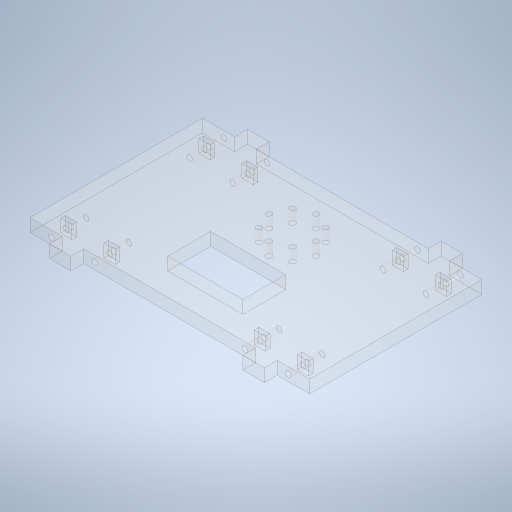
# Autodesk Inventor part: frame_waist_frames_linker1
Saved by Autodesk Inventor 2024 (Build 280153000, 153)
## iProperties
Created: 2024-09-07
Part Number: frame_waist_frames_linker1
Material: PMMA 플라스틱
Document SubType Name: Modeling
Designer: jmha0
Density: 1.188 g/cm^3
Appearance: 폴리카보네이트 - 선명
Author: jmha0
Autodesk Inventor part; units mm, degrees
ref_plane "YZ Plane" through (0, 0, 0) normal (1, 0, 0) x (0, 1, 0)
ref_plane "XZ Plane" through (0, 0, 0) normal (0, 1, 0) x (-1, 0, 0)
ref_plane "XY Plane" through (0, 0, 0) normal (0, 0, 1) x (1, 0, 0)
sketch "스케치1" plane through (0, 0, 0) normal (0, 1, 0) x (-1, 0, 0)
  circle A0 centre (21.5232, -91.3038) radius 1.65
  circle A1 centre (37.0796, -75.7475) radius 1.65
  circle A2 centre (29.3014, -72.5257) radius 1.65
  circle A3 centre (29.3014, -94.5257) radius 1.65
  circle A4 centre (18.3014, -83.5257) radius 1.65
  circle A5 centre (40.3014, -83.5257) radius 1.65
  circle A6 centre (21.5232, -75.7475) radius 1.65
  circle A7 centre (37.0796, -91.3038) radius 1.65
  line L0 (-35.8986, -112.7138) -> (94.5014, -112.7138)
  line L1 (94.5014, -112.7138) -> (94.5014, -20.3138)
  line L2 (94.5014, -20.3138) -> (-35.8986, -20.3138)
  line L3 (-35.8986, -20.3138) -> (-35.8986, -112.7138)
  circle A8 centre (-5.7486, -109.7138) radius 1.45
  circle A9 centre (-25.8486, -109.7138) radius 1.45
  circle A10 centre (-25.8486, -23.3138) radius 1.45
  circle A11 centre (-5.7486, -23.3138) radius 1.45
  circle A12 centre (64.3514, -23.3138) radius 1.45
  circle A13 centre (84.4514, -23.3138) radius 1.45
  circle A14 centre (84.4514, -109.7138) radius 1.45
  circle A15 centre (64.3514, -109.7138) radius 1.45
  line L4 (94.5014, -20.3138) -> (-35.8986, -20.3138)
  line L5 (-35.8986, -20.3138) -> (-35.8986, -26.3138)
  line L6 (-35.8986, -26.3138) -> (94.5014, -26.3138)
  line L7 (94.5014, -26.3138) -> (94.5014, -20.3138)
  line L8 (94.5014, -112.7138) -> (-35.8986, -112.7138)
  line L9 (-35.8986, -112.7138) -> (-35.8986, -106.7138)
  line L10 (-35.8986, -106.7138) -> (94.5014, -106.7138)
  line L11 (94.5014, -106.7138) -> (94.5014, -112.7138)
  circle A16 centre (29.3014, -94.5257) radius 1.35
  circle A17 centre (21.5232, -91.3038) radius 1.35
  circle A18 centre (18.3014, -83.5257) radius 1.35
  circle A19 centre (21.5232, -75.7475) radius 1.35
  circle A20 centre (29.3014, -72.5257) radius 1.35
  circle A21 centre (37.0796, -75.7475) radius 1.35
  circle A22 centre (40.3014, -83.5257) radius 1.35
  circle A23 centre (37.0796, -91.3038) radius 1.35
  point P0 (0, 0)
  point P1 (81.123, -83.5257)
  dimension "d0" = 6
  dimension "d1" = 6
  dimension "d16" = 2.7
  dimension "d17" = 2.7
  dimension "d18" = 2.7
  dimension "d19" = 2.7
  dimension "d20" = 2.7
  dimension "d21" = 2.7
  dimension "d22" = 2.7
  dimension "d23" = 2.7
  constraints: 24 centre point, 24 end point, 8 coincident, 4 parallel, 2 horizontal, 2 perpendicular, 2 point on line
  measures "d0" distance of L5.end L4.end
  measures "d1" distance of L8.end L9.end
  measures "d16" diameter of A16
  measures "d17" diameter of A17
  measures "d18" diameter of A18
  measures "d19" diameter of A19
  measures "d20" diameter of A20
  measures "d21" diameter of A21
  measures "d22" diameter of A22
  measures "d23" diameter of A23
extrude "돌출1" add sketch "스케치1" along normal blind 6 contours A0 | A1 | A2 | A3 | A4 | A5 | A6 | A7 | L3 L6 L1 L10
sketch "스케치2" plane through (-94.5014, 0, -26.3138) normal (0, 0, 1) x (1, 0, 0)
  line L0 (0, 0) -> (130.4, 0) projected
  line L1 (130.4, 0) -> (130.4, 6) projected
  line L2 (0, 6) -> (130.4, 6) projected
  line L3 (0, 0) -> (0, 6) projected
  line L4 (0, 6) -> (10.05, 6)
  line L5 (10.05, 6) -> (30.15, 6)
  line L6 (130.4, 6) -> (120.35, 6)
  line L7 (130.4, 6) -> (0, 6) projected
  line L8 (120.35, 6) -> (100.25, 6)
  circle A0 centre (10.05, 3) radius 1.35
  circle A1 centre (30.15, 3) radius 1.35
  circle A2 centre (100.25, 3) radius 1.35
  circle A3 centre (120.35, 3) radius 1.35
  point P0 (94.5014, 0)
  dimension "d4" = 10.05
  dimension "d5" = 20.1
  dimension "d6" = 10.05
  dimension "d7" = 20.1
  dimension "d8" = 2.7
  dimension "d9" = 2.7
  dimension "d10" = 2.7
  dimension "d11" = 2.7
  constraints: 8 end point, 4 centre point, 4 point on line
  measures "d4" distance of L2.start L4.end
  measures "d5" distance of L4.end L5.end
  measures "d6" distance of L1.end L6.end
  measures "d7" distance of L6.end L8.end
  measures "d8" diameter of A0
  measures "d9" diameter of A1
  measures "d10" diameter of A2
  measures "d11" diameter of A3
extrude "돌출2" cut sketch "스케치2" against normal blind 16 contours A0 | A1 | A2 | A3
sketch "스케치3" plane through (35.8986, 0, -106.7138) normal (0, 0, -1) x (-1, 0, 0)
  circle A0 centre (30.15, 3) radius 1.35 projected
  circle A1 centre (100.25, 3) radius 1.35 projected
  point P0 (35.8986, 0)
extrude "돌출3" cut sketch "스케치3" against normal blind 16
sketch "스케치4" plane through (35.8986, 0, -106.7138) normal (0, 0, -1) x (-1, 0, 0)
  circle A0 centre (10.05, 3) radius 1.35 projected
  circle A1 centre (120.35, 3) radius 1.35 projected
  point P0 (35.8986, 0)
extrude "돌출4" cut sketch "스케치4" against normal blind 16
sketch "스케치5" plane through (0, 6, 0) normal (0, 1, 0) x (1, 0, 0)
  circle A0 centre (-18.3014, 83.5257) radius 1.35 projected
  circle A1 centre (-18.3014, 83.5257) radius 1.35 projected
  circle A2 centre (-18.3014, 83.5257) radius 1.35 projected
  circle A3 centre (-18.3014, 83.5257) radius 1.35 projected
  circle A4 centre (-21.5232, 91.3038) radius 1.35 projected
  circle A5 centre (-21.5232, 91.3038) radius 1.35 projected
  circle A6 centre (-21.5232, 91.3038) radius 1.35 projected
  line L0 (35.8986, 106.7138) -> (-94.5014, 106.7138) projected
  line L1 (35.8986, 106.7138) -> (-94.5014, 106.7138) projected
  line L2 (-85.8014, 106.7138) -> (-83.1014, 106.7138) projected
  line L3 (24.4986, 106.7138) -> (27.1986, 106.7138) projected
  line L4 (-65.7014, 106.7138) -> (-63.0014, 106.7138) projected
  line L5 (4.3986, 106.7138) -> (7.0986, 106.7138) projected
  line L6 (35.8986, 106.7138) -> (-94.5014, 106.7138) projected
  line L7 (35.8986, 106.7138) -> (-94.5014, 106.7138) projected
  line L8 (-94.5014, 106.7138) -> (-94.5014, 26.3138) projected
  line L9 (-94.5014, 26.3138) -> (35.8986, 26.3138) projected
  line L10 (35.8986, 26.3138) -> (35.8986, 106.7138) projected
  line L11 (35.8986, 106.7138) -> (-94.5014, 106.7138) projected
  circle A7 centre (-40.3014, 83.5257) radius 1.35 projected
  circle A8 centre (-37.0796, 91.3038) radius 1.35 projected
  circle A9 centre (-29.3014, 94.5257) radius 1.35 projected
  circle A10 centre (-21.5232, 91.3038) radius 1.35 projected
  circle A11 centre (-18.3014, 83.5257) radius 1.35 projected
  circle A12 centre (-21.5232, 75.7475) radius 1.35 projected
  circle A13 centre (-29.3014, 72.5257) radius 1.35 projected
  circle A14 centre (-37.0796, 75.7475) radius 1.35 projected
  line L12 (-94.5014, 106.7138) -> (-94.5014, 26.3138) projected
  line L13 (35.8986, 106.7138) -> (-94.5014, 106.7138) projected
  line L14 (35.8986, 26.3138) -> (35.8986, 106.7138) projected
  line L15 (-94.5014, 26.3138) -> (35.8986, 26.3138) projected
  circle A15 centre (-40.3014, 83.5257) radius 1.35 projected
  circle A16 centre (-37.0796, 91.3038) radius 1.35 projected
  circle A17 centre (-29.3014, 94.5257) radius 1.35 projected
  circle A18 centre (-21.5232, 91.3038) radius 1.35 projected
  circle A19 centre (-18.3014, 83.5257) radius 1.35 projected
  circle A20 centre (-21.5232, 75.7475) radius 1.35 projected
  circle A21 centre (-29.3014, 72.5257) radius 1.35 projected
  circle A22 centre (-37.0796, 75.7475) radius 1.35 projected
  circle A23 centre (-29.3014, 72.5257) radius 1.35 projected
  circle A24 centre (-29.3014, 72.5257) radius 1.35 projected
  circle A25 centre (-29.3014, 72.5257) radius 1.35 projected
  circle A26 centre (-37.0796, 91.3038) radius 1.35 projected
  circle A27 centre (-37.0796, 91.3038) radius 1.35 projected
  circle A28 centre (-37.0796, 91.3038) radius 1.35 projected
  circle A29 centre (-40.3014, 83.5257) radius 1.35 projected
  circle A30 centre (-40.3014, 83.5257) radius 1.35 projected
  circle A31 centre (-40.3014, 83.5257) radius 1.35 projected
  circle A32 centre (-40.3014, 83.5257) radius 1.35 projected
  line L16 (-65.7014, 106.7138) -> (-63.0014, 106.7138) projected
  line L17 (-94.5014, 106.7138) -> (-94.5014, 26.3138) projected
  line L18 (-85.8014, 90.7138) -> (-83.1014, 90.7138) projected
  line L19 (-85.8014, 90.7138) -> (-83.1014, 90.7138) projected
  line L20 (-85.8014, 90.7138) -> (-83.1014, 90.7138) projected
  line L21 (-85.8014, 106.7138) -> (-83.1014, 106.7138) projected
  line L22 (-85.8014, 106.7138) -> (-83.1014, 106.7138) projected
  circle A33 centre (-37.0796, 91.3038) radius 1.35 projected
  line L23 (-94.5014, 26.3138) -> (35.8986, 26.3138) projected
  line L24 (7.0986, 26.3138) -> (4.3986, 26.3138) projected
  line L25 (-63.0014, 26.3138) -> (-65.7014, 26.3138) projected
  line L26 (27.1986, 26.3138) -> (24.4986, 26.3138) projected
  line L27 (-83.1014, 26.3138) -> (-85.8014, 26.3138) projected
  line L28 (-94.5014, 26.3138) -> (35.8986, 26.3138) projected
  line L29 (-94.5014, 26.3138) -> (35.8986, 26.3138) projected
  line L30 (-94.5014, 26.3138) -> (35.8986, 26.3138) projected
  line L31 (4.3986, 106.7138) -> (7.0986, 106.7138) projected
  line L32 (24.4986, 90.7138) -> (27.1986, 90.7138) projected
  line L33 (24.4986, 90.7138) -> (27.1986, 90.7138) projected
  line L34 (24.4986, 90.7138) -> (27.1986, 90.7138) projected
  line L35 (24.4986, 106.7138) -> (27.1986, 106.7138) projected
  line L36 (24.4986, 106.7138) -> (27.1986, 106.7138) projected
  line L37 (35.8986, 26.3138) -> (35.8986, 106.7138) projected
  line L38 (35.8986, 26.3138) -> (35.8986, 106.7138) projected
  line L39 (-63.0014, 42.3138) -> (-65.7014, 42.3138) projected
  line L40 (-63.0014, 42.3138) -> (-65.7014, 42.3138) projected
  circle A34 centre (-29.3014, 72.5257) radius 1.35 projected
  circle A35 centre (-29.3014, 94.5257) radius 1.35 projected
  circle A36 centre (-29.3014, 94.5257) radius 1.35 projected
  circle A37 centre (-29.3014, 94.5257) radius 1.35 projected
  circle A38 centre (-29.3014, 94.5257) radius 1.35 projected
  circle A39 centre (-21.5232, 75.7475) radius 1.35 projected
  circle A40 centre (-21.5232, 75.7475) radius 1.35 projected
  circle A41 centre (-21.5232, 75.7475) radius 1.35 projected
  circle A42 centre (-21.5232, 75.7475) radius 1.35 projected
  circle A43 centre (-21.5232, 91.3038) radius 1.35 projected
  line L41 (-63.0014, 26.3138) -> (-65.7014, 26.3138) projected
  line L42 (-63.0014, 42.3138) -> (-65.7014, 42.3138) projected
  line L43 (-63.0014, 26.3138) -> (-65.7014, 26.3138) projected
  line L44 (-83.1014, 26.3138) -> (-85.8014, 26.3138) projected
  line L45 (-83.1014, 42.3138) -> (-85.8014, 42.3138) projected
  line L46 (-83.1014, 26.3138) -> (-85.8014, 26.3138) projected
  line L47 (-94.5014, 106.7138) -> (-94.5014, 26.3138) projected
  line L48 (-94.5014, 106.7138) -> (-94.5014, 26.3138) projected
  line L49 (-94.5014, 106.7138) -> (-94.5014, 26.3138) projected
  circle A44 centre (-37.0796, 75.7475) radius 1.35 projected
  circle A45 centre (-37.0796, 75.7475) radius 1.35 projected
  circle A46 centre (-37.0796, 75.7475) radius 1.35 projected
  circle A47 centre (-37.0796, 75.7475) radius 1.35 projected
  line L50 (-65.7014, 90.7138) -> (-63.0014, 90.7138) projected
  line L51 (-65.7014, 90.7138) -> (-63.0014, 90.7138) projected
  line L52 (-65.7014, 106.7138) -> (-63.0014, 106.7138) projected
  line L53 (-65.7014, 90.7138) -> (-63.0014, 90.7138) projected
  line L54 (-83.1014, 42.3138) -> (-85.8014, 42.3138) projected
  line L55 (-83.1014, 42.3138) -> (-85.8014, 42.3138) projected
  line L56 (27.1986, 42.3138) -> (24.4986, 42.3138) projected
  line L57 (27.1986, 26.3138) -> (24.4986, 26.3138) projected
  line L58 (7.0986, 26.3138) -> (4.3986, 26.3138) projected
  line L59 (7.0986, 42.3138) -> (4.3986, 42.3138) projected
  line L60 (4.3986, 90.7138) -> (7.0986, 90.7138) projected
  line L61 (7.0986, 42.3138) -> (4.3986, 42.3138) projected
  line L62 (7.0986, 42.3138) -> (4.3986, 42.3138) projected
  line L63 (7.0986, 26.3138) -> (4.3986, 26.3138) projected
  line L64 (4.3986, 90.7138) -> (7.0986, 90.7138) projected
  line L65 (4.3986, 90.7138) -> (7.0986, 90.7138) projected
  line L66 (4.3986, 106.7138) -> (7.0986, 106.7138) projected
  line L67 (35.8986, 26.3138) -> (35.8986, 106.7138) projected
  line L68 (35.8986, 26.3138) -> (35.8986, 106.7138) projected
  line L69 (27.1986, 42.3138) -> (24.4986, 42.3138) projected
  line L70 (27.1986, 26.3138) -> (24.4986, 26.3138) projected
  line L71 (27.1986, 42.3138) -> (24.4986, 42.3138) projected
  line L72 (27.1986, 26.3138) -> (27.1986, 42.3138) projected
  line L73 (24.4986, 26.3138) -> (24.4986, 42.3138) projected
  line L74 (7.0986, 26.3138) -> (7.0986, 42.3138) projected
  line L75 (4.3986, 26.3138) -> (4.3986, 42.3138) projected
  line L76 (-63.0014, 26.3138) -> (-63.0014, 42.3138) projected
  line L77 (-85.8014, 26.3138) -> (-85.8014, 42.3138) projected
  line L78 (-83.1014, 26.3138) -> (-83.1014, 42.3138) projected
  line L79 (-65.7014, 26.3138) -> (-65.7014, 42.3138) projected
  line L80 (-63.0014, 106.7138) -> (-63.0014, 90.7138) projected
  line L81 (-65.7014, 106.7138) -> (-65.7014, 90.7138) projected
  line L82 (-83.1014, 106.7138) -> (-83.1014, 90.7138) projected
  line L83 (-85.8014, 106.7138) -> (-85.8014, 90.7138) projected
  line L84 (4.3986, 106.7138) -> (4.3986, 90.7138) projected
  line L85 (7.0986, 106.7138) -> (7.0986, 90.7138) projected
  line L86 (24.4986, 106.7138) -> (24.4986, 90.7138) projected
  line L87 (27.1986, 106.7138) -> (27.1986, 90.7138) projected
  line L88 (28.4486, 99.8138) -> (23.2486, 99.8138)
  line L89 (23.2486, 99.8138) -> (23.2486, 97.6138)
  line L90 (23.2486, 97.6138) -> (28.4486, 97.6138)
  line L91 (28.4486, 97.6138) -> (28.4486, 99.8138)
  line L92 (28.4486, 99.8138) -> (23.2486, 97.6138) construction
  line L93 (23.2486, 99.8138) -> (28.4486, 97.6138) construction
  line L94 (8.3486, 99.8138) -> (3.1486, 99.8138)
  line L95 (3.1486, 99.8138) -> (3.1486, 97.6138)
  line L96 (3.1486, 97.6138) -> (8.3486, 97.6138)
  line L97 (8.3486, 97.6138) -> (8.3486, 99.8138)
  line L98 (8.3486, 99.8138) -> (3.1486, 97.6138) construction
  line L99 (3.1486, 99.8138) -> (8.3486, 97.6138) construction
  line L100 (-61.7514, 96.5138) -> (-66.9514, 98.7138) construction
  line L101 (-66.9514, 96.5138) -> (-61.7514, 98.7138) construction
  line L102 (-81.8514, 99.8138) -> (-87.0514, 99.8138)
  line L103 (-87.0514, 99.8138) -> (-87.0514, 97.6138)
  line L104 (-87.0514, 97.6138) -> (-81.8514, 97.6138)
  line L105 (-81.8514, 97.6138) -> (-81.8514, 99.8138)
  line L106 (-81.8514, 99.8138) -> (-87.0514, 97.6138) construction
  line L107 (-87.0514, 99.8138) -> (-81.8514, 97.6138) construction
  line L108 (-61.7514, 99.8138) -> (-66.9514, 99.8138)
  line L109 (-66.9514, 99.8138) -> (-66.9514, 97.6138)
  line L110 (-66.9514, 97.6138) -> (-61.7514, 97.6138)
  line L111 (-61.7514, 97.6138) -> (-61.7514, 99.8138)
  line L112 (-61.7514, 99.8138) -> (-66.9514, 97.6138) construction
  line L113 (-66.9514, 99.8138) -> (-61.7514, 97.6138) construction
  line L114 (-81.8514, 35.4138) -> (-87.0514, 35.4138)
  line L115 (-87.0514, 35.4138) -> (-87.0514, 33.2138)
  line L116 (-87.0514, 33.2138) -> (-81.8514, 33.2138)
  line L117 (-81.8514, 33.2138) -> (-81.8514, 35.4138)
  line L118 (-81.8514, 35.4138) -> (-87.0514, 33.2138) construction
  line L119 (-87.0514, 35.4138) -> (-81.8514, 33.2138) construction
  line L120 (-61.7514, 35.4138) -> (-66.9514, 35.4138)
  line L121 (-66.9514, 35.4138) -> (-66.9514, 33.2138)
  line L122 (-66.9514, 33.2138) -> (-61.7514, 33.2138)
  line L123 (-61.7514, 33.2138) -> (-61.7514, 35.4138)
  line L124 (-61.7514, 35.4138) -> (-66.9514, 33.2138) construction
  line L125 (-66.9514, 35.4138) -> (-61.7514, 33.2138) construction
  line L126 (8.3486, 35.4138) -> (3.1486, 35.4138)
  line L127 (3.1486, 35.4138) -> (3.1486, 33.2138)
  line L128 (3.1486, 33.2138) -> (8.3486, 33.2138)
  line L129 (8.3486, 33.2138) -> (8.3486, 35.4138)
  line L130 (8.3486, 35.4138) -> (3.1486, 33.2138) construction
  line L131 (3.1486, 35.4138) -> (8.3486, 33.2138) construction
  line L132 (28.4486, 35.4138) -> (23.2486, 35.4138)
  line L133 (23.2486, 35.4138) -> (23.2486, 33.2138)
  line L134 (23.2486, 33.2138) -> (28.4486, 33.2138)
  line L135 (28.4486, 33.2138) -> (28.4486, 35.4138)
  line L136 (28.4486, 35.4138) -> (23.2486, 33.2138) construction
  line L137 (23.2486, 35.4138) -> (28.4486, 33.2138) construction
  point P0 (0, 0)
  point P1 (25.8486, 98.7138)
  point P2 (5.7486, 98.7138)
  point P3 (-64.3514, 97.6138)
  point P4 (-84.4514, 98.7138)
  point P5 (-64.3514, 98.7138)
  point P6 (-84.4514, 34.3138)
  point P7 (-64.3514, 34.3138)
  point P8 (5.7486, 34.3138)
  point P9 (25.8486, 34.3138)
  dimension "d26" = 5.2
  dimension "d27" = 2.2
  dimension "d28" = 5.2
  dimension "d29" = 2.2
  dimension "d30" = 5.2
  dimension "d31" = 2.2
  dimension "d32" = 5.2
  dimension "d33" = 2.2
  dimension "d34" = 5.2
  dimension "d35" = 2.2
  dimension "d36" = 5.2
  dimension "d37" = 2.2
  dimension "d38" = 5.2
  dimension "d39" = 2.2
  dimension "d40" = 5.2
  dimension "d41" = 2.2
  constraints: 100 end point, 18 midpoint, 16 parallel, 8 horizontal, 8 perpendicular, 3 point on line, 6 other
  measures "d26" distance of L90.end L89.end
  measures "d27" distance of L89.end L88.end
  measures "d28" distance of L96.end L95.end
  measures "d29" distance of L95.end L94.end
  measures "d30" distance of L100.end L101.end
  measures "d31" distance of L101.start L100.end
  measures "d32" distance of L104.end L103.end
  measures "d33" distance of L103.end L102.end
  measures "d34" distance of L110.end L109.end
  measures "d35" distance of L109.end L108.end
  measures "d36" distance of L116.end L115.end
  measures "d37" distance of L115.end L114.end
  measures "d38" distance of L128.end L127.end
  measures "d39" distance of L127.end L126.end
  measures "d40" distance of L134.end L133.end
  measures "d41" distance of L133.end L132.end
extrude "돌출5" cut sketch "스케치5" against normal blind 16 contours L88 L91 L90 L87 | L87 L90 L86 L88 | L86 L90 L89 L88 | L134 L73 L132 L72 | L72 L132 L135 L134 | L94 L97 L96 L85 | L85 L96 L84 L94 | L134 L133 L132 L73 | L84 L96 L95 L94 | L128 L75 L126 L74 | L74 L126 L129 L128 | L108 L111 L110 L80 | L80 L110 L81 L108 | L128 L127 L126 L75 | L81 L110 L109 L108 | L122 L79 L120 L76 | L76 L120 L123 L122 | L102 L105 L104 L82 | L82 L104 L83 L102 | L122 L121 L120 L79 | L83 L104 L103 L102 | L116 L77 L114 L78 | L78 L114 L117 L116 | L116 L115 L114 L77
sketch "스케치6" plane through (0, 6, 0) normal (0, 1, 0) x (1, 0, 0)
  line L0 (23.2486, 97.6138) -> (23.2486, 99.8138) projected
  line L1 (23.2486, 99.8138) -> (28.4486, 99.8138) projected
  line L2 (28.4486, 99.8138) -> (28.4486, 97.6138) projected
  line L3 (28.4486, 97.6138) -> (23.2486, 97.6138) projected
  line L4 (-66.9514, 33.2138) -> (-66.9514, 35.4138) projected
  line L5 (-66.9514, 35.4138) -> (-61.7514, 35.4138) projected
  line L6 (-61.7514, 35.4138) -> (-61.7514, 33.2138) projected
  line L7 (-61.7514, 33.2138) -> (-66.9514, 33.2138) projected
  line L8 (-87.0514, 97.6138) -> (-87.0514, 99.8138) projected
  line L9 (-87.0514, 99.8138) -> (-81.8514, 99.8138) projected
  line L10 (-81.8514, 99.8138) -> (-81.8514, 97.6138) projected
  line L11 (-81.8514, 97.6138) -> (-87.0514, 97.6138) projected
  line L12 (3.1486, 33.2138) -> (3.1486, 35.4138) projected
  line L13 (3.1486, 35.4138) -> (8.3486, 35.4138) projected
  line L14 (8.3486, 35.4138) -> (8.3486, 33.2138) projected
  line L15 (8.3486, 33.2138) -> (3.1486, 33.2138) projected
  line L16 (3.1486, 97.6138) -> (3.1486, 99.8138) projected
  line L17 (3.1486, 99.8138) -> (8.3486, 99.8138) projected
  line L18 (8.3486, 99.8138) -> (8.3486, 97.6138) projected
  line L19 (8.3486, 97.6138) -> (3.1486, 97.6138) projected
  line L20 (-87.0514, 33.2138) -> (-87.0514, 35.4138) projected
  line L21 (-87.0514, 35.4138) -> (-81.8514, 35.4138) projected
  line L22 (-81.8514, 35.4138) -> (-81.8514, 33.2138) projected
  line L23 (-81.8514, 33.2138) -> (-87.0514, 33.2138) projected
  line L24 (-66.9514, 97.6138) -> (-66.9514, 99.8138) projected
  line L25 (-66.9514, 99.8138) -> (-61.7514, 99.8138) projected
  line L26 (-61.7514, 99.8138) -> (-61.7514, 97.6138) projected
  line L27 (-61.7514, 97.6138) -> (-66.9514, 97.6138) projected
  line L28 (23.2486, 33.2138) -> (23.2486, 35.4138) projected
  line L29 (23.2486, 35.4138) -> (28.4486, 35.4138) projected
  line L30 (28.4486, 35.4138) -> (28.4486, 33.2138) projected
  line L31 (28.4486, 33.2138) -> (23.2486, 33.2138) projected
  line L32 (-94.5014, 106.7138) -> (-94.5014, 26.3138) projected
  line L33 (-94.5014, 26.3138) -> (35.8986, 26.3138) projected
  line L34 (35.8986, 26.3138) -> (35.8986, 106.7138) projected
  line L35 (35.8986, 106.7138) -> (-94.5014, 106.7138) projected
  circle A0 centre (-40.3014, 83.5257) radius 1.35 projected
  circle A1 centre (-37.0796, 91.3038) radius 1.35 projected
  circle A2 centre (-29.3014, 94.5257) radius 1.35 projected
  circle A3 centre (-21.5232, 91.3038) radius 1.35 projected
  circle A4 centre (-18.3014, 83.5257) radius 1.35 projected
  circle A5 centre (-21.5232, 75.7475) radius 1.35 projected
  circle A6 centre (-29.3014, 72.5257) radius 1.35 projected
  circle A7 centre (-37.0796, 75.7475) radius 1.35 projected
  line L36 (-11.8014, 62.8931) -> (-46.8014, 62.8931)
  line L37 (-46.8014, 62.8931) -> (-46.8014, 42.8931)
  line L38 (-46.8014, 42.8931) -> (-11.8014, 42.8931)
  line L39 (-11.8014, 42.8931) -> (-11.8014, 62.8931)
  line L40 (-11.8014, 62.8931) -> (-46.8014, 42.8931) construction
  line L41 (-46.8014, 62.8931) -> (-11.8014, 42.8931) construction
  point P0 (0, 0)
  point P1 (-29.3014, 52.8931)
  dimension "d44" = 35
  dimension "d45" = 20
  constraints: 12 end point, 2 midpoint, 2 parallel, 1 horizontal, 1 perpendicular
  measures "d44" distance of L36.start L36.end
  measures "d45" distance of L37.end L36.end
extrude "돌출6" cut sketch "스케치6" against normal blind 10 contours L39 L38 L37 L36
sketch "스케치7" plane through (-94.5014, 0, -26.3138) normal (0, 0, 1) x (1, 0, 0)
  circle A0 centre (100.25, 3) radius 1.35 projected
  circle A1 centre (30.15, 3) radius 1.35 projected
  circle A2 centre (120.35, 3) radius 1.35 projected
  circle A3 centre (10.05, 3) radius 1.35 projected
  line L0 (0, 0) -> (130.4, 0) projected
  line L1 (130.4, 0) -> (130.4, 6) projected
  line L2 (0, 6) -> (130.4, 6) projected
  line L3 (0, 0) -> (0, 6) projected
  line L4 (12.65, 6) -> (12.65, 0) projected
  line L5 (27.55, 6) -> (27.55, 0) projected
  line L6 (102.85, 6) -> (102.85, 0) projected
  line L7 (117.75, 6) -> (117.75, 0) projected
  line L8 (27.55, 3) -> (20.1, 3)
  line L9 (25.1, 0) -> (25.1, 6)
  line L10 (25.1, 6) -> (15.1, 6)
  line L11 (15.1, 6) -> (15.1, 0)
  line L12 (15.1, 0) -> (25.1, 0)
  line L13 (25.1, 0) -> (15.1, 6) construction
  line L14 (25.1, 6) -> (15.1, 0) construction
  line L15 (102.85, 3) -> (110.3, 3)
  line L16 (105.3, 0) -> (105.3, 6)
  line L17 (105.3, 6) -> (115.3, 6)
  line L18 (115.3, 6) -> (115.3, 0)
  line L19 (115.3, 0) -> (105.3, 0)
  line L20 (105.3, 0) -> (115.3, 6) construction
  line L21 (105.3, 6) -> (115.3, 0) construction
  point P0 (94.5014, 0)
  point P1 (12.65, 3)
  dimension "d48" = 14.9
  dimension "d49" = 7.45
  dimension "d50" = 10
  dimension "d51" = 7.45
  dimension "d52" = 10
  constraints: 28 end point, 7 midpoint, 5 parallel, 4 perpendicular, 1 horizontal
  measures "d48" distance of L8.start point (12.65, 3)
  measures "d49" distance of L8.start L8.end
  measures "d50" distance of L10.end L9.end
  measures "d51" distance of L15.start L15.end
  measures "d52" distance of L16.end L17.end
extrude "돌출7" add sketch "스케치7" along normal blind 6 contours L11 L2 L9 L0 | L16 L2 L18 L0
sketch "스케치8" plane through (35.8986, 0, -106.7138) normal (0, 0, -1) x (-1, 0, 0)
  line L0 (0, 6) -> (130.4, 6) projected
  circle A0 centre (120.35, 3) radius 1.35 projected
  circle A1 centre (10.05, 3) radius 1.35 projected
  circle A2 centre (100.25, 3) radius 1.35 projected
  circle A3 centre (30.15, 3) radius 1.35 projected
  line L1 (0, 0) -> (130.4, 0) projected
  line L2 (130.4, 0) -> (130.4, 6) projected
  line L3 (0, 6) -> (130.4, 6) projected
  line L4 (0, 0) -> (0, 6) projected
  line L5 (15.1, 6) -> (15.1, 0) projected
  line L6 (25.1, 0) -> (25.1, 6) projected
  line L7 (115.3, 0) -> (115.3, 6) projected
  line L8 (105.3, 6) -> (105.3, 0) projected
  point P0 (35.8986, 0)
extrude "돌출8" add sketch "스케치8" along normal blind 6 contours L0 L6 L1 L5 | L0 L7 L1 L8
